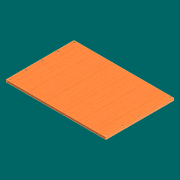
# Autodesk Inventor part: sideFace
Saved by Autodesk Inventor 2016 SP1 (Build 200210100, 210)
## iProperties
Created: 2016-04-01
Part Number: sideFace
Material: Wood (Cherry)
Document SubType Name: Modeling
Designer: sawai
Density: 0.63 g/cm^3
Appearance: Cherry - Natural Low Gloss
Author: sawai
Autodesk Inventor part; units mm, degrees
ref_plane "YZ Plane" through (0, 0, 0) normal (1, 0, 0) x (0, 1, 0)
ref_plane "XZ Plane" through (0, 0, 0) normal (0, 1, 0) x (-1, 0, 0)
ref_plane "XY Plane" through (0, 0, 0) normal (0, 0, 1) x (1, 0, 0)
sketch "Sketch1" plane through (0, 0, 0) normal (0, 1, 0) x (-1, 0, 0)
  line L0 (170, 250) -> (-170, 250)
  line L1 (-170, 250) -> (-170, -250)
  line L2 (-170, -250) -> (170, -250)
  line L3 (170, -250) -> (170, 250)
  line L4 (170, 250) -> (-170, -250) construction
  line L5 (-170, 250) -> (170, -250) construction
  point P0 (0, 0)
  dimension "d0" = 340
  dimension "d1" = 500
  constraints: 12 end point, 2 midpoint, 2 parallel, 1 horizontal, 1 perpendicular
  measures "d0" distance of L2.end L1.end
  measures "d1" distance between parallel lines of L0 L2
extrude "Extrusion1" add sketch "Sketch1" along normal blind 11.1125
sketch "Sketch2" plane through (0, 11.1125, 0) normal (0, 1, 0) x (1, 0, 0)
  line L0 (-170, -250) -> (170, -250) projected
  line L1 (170, -250) -> (170, 250) projected
  line L2 (170, 250) -> (-170, 250) projected
  line L3 (-170, 250) -> (-170, -250) projected
  point P0 (0, 0)
  point P1 (-160, -240)
  dimension "d4" = 10
  dimension "d5" = 10
  measures "d4" distance from line of L3 point (-160, -240)
  measures "d5" distance from line of L0 point (-160, -240)
hole "Hole1" at (-160, 11.1125, 240) direction (0, -1, 0) diameter 5.5 end through all counterbore diameter 10 counterbore depth 5 clearance for "Socket Head Cap Screw" size "M5" standard "Ansi Metric M Profile"
pattern_linear "Rectangular Pattern1" count 2 spacing 480 along (0, 0, -1) count 5 spacing 80 along (1, 0, 0) of "Hole1"
sketch "Sketch3" plane through (-170, 0, -250) normal (-1, 0, 0) x (0, 0, 1)
  line L0 (0, 0) -> (500, 0) projected
  line L1 (500, 0) -> (500, 11.1125) projected
  line L2 (0, 11.1125) -> (500, 11.1125) projected
  line L3 (0, 0) -> (0, 11.1125) projected
  line L4 (0, 0) -> (0, 11.1125) projected
  arc A0 (0, 3.175) -> (0, 6.35) centre (0, 4.7625) ccw
  point P0 (250, 0)
  dimension "d19" = 1.5875
  dimension "d20" = 6.35
  constraints: 3 point on line, 2 point on circle, 1 centre point
  measures "d19" radius of A0
  measures "d20" distance from line of L2 A0.centre
extrude "oRingGroove" cut sketch "Sketch3" against normal through all contours L3 A0
mirror "Mirror1" about plane through (0, 0, 0) normal (0, 0, 1) of "oRingGroove"
equation "\"d1\" = depth"
equation "\"d2\" = facingThickness - facingGasketThickness"
equation "\"d19\" = 0.125 * facingThickness"
equation "\"d20\" = 0.5 * facingThickness"
equation "\"depth\" = 500"
equation "\"facingThickness\" = 12.7"
equation "\"facingGasketThickness\" = 1.5875"
body "Solid1"
